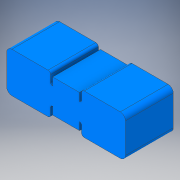
# Autodesk Inventor part: Connecter EM
Saved by Autodesk Inventor 2017 (Build 210142000, 142)
## iProperties
Created: 2020-02-07
Part Number: Connecter EM
Material: ABS Plastic
Document SubType Name: Modeling
Designer: 10042265
Density: 1.06 g/cm^3
Appearance: Smooth - White
Author: 10042265
Autodesk Inventor part; units mm, degrees
ref_plane "YZ Plane" through (0, 0, 0) normal (1, 0, 0) x (0, 1, 0)
ref_plane "XZ Plane" through (0, 0, 0) normal (0, 1, 0) x (-1, 0, 0)
ref_plane "XY Plane" through (0, 0, 0) normal (0, 0, 1) x (1, 0, 0)
sketch "Sketch1" plane through (0, 0, 0) normal (0, 0, 1) x (1, 0, 0)
  line L0 (-29.21, 0) -> (-29.21, 7.366)
  line L1 (-26.67, 9.906) -> (-8.89, 9.906)
  line L2 (-7.62, 8.636) -> (-7.62, 5.334)
  line L3 (-6.604, 4.318) -> (-6.604, 4.318)
  line L4 (-6.604, 4.318) -> (-6.604, 8.128)
  line L5 (-6.604, 8.128) -> (0, 8.128)
  arc A0 (-26.67, 9.906) -> (-29.21, 7.366) centre (-26.67, 7.366) ccw
  arc A1 (-7.62, 8.636) -> (-8.89, 9.906) centre (-8.89, 8.636) ccw
  arc A2 (-7.62, 5.334) -> (-6.604, 4.318) centre (-6.604, 5.334) ccw
  line L6 (29.21, 0) -> (29.21, 7.366)
  line L7 (26.67, 9.906) -> (8.89, 9.906)
  line L8 (7.62, 8.636) -> (7.62, 5.334)
  line L9 (6.604, 4.318) -> (6.604, 4.318)
  line L10 (6.604, 4.318) -> (6.604, 8.128)
  line L11 (6.604, 8.128) -> (0, 8.128)
  arc A3 (29.21, 7.366) -> (26.67, 9.906) centre (26.67, 7.366) ccw
  arc A4 (8.89, 9.906) -> (7.62, 8.636) centre (8.89, 8.636) ccw
  arc A5 (6.604, 4.318) -> (7.62, 5.334) centre (6.604, 5.334) ccw
  line L12 (-29.21, 0) -> (-29.21, -7.366)
  line L13 (-26.67, -9.906) -> (-8.89, -9.906)
  line L14 (-7.62, -8.636) -> (-7.62, -5.334)
  arc A6 (-29.21, -7.366) -> (-26.67, -9.906) centre (-26.67, -7.366) ccw
  arc A7 (-8.89, -9.906) -> (-7.62, -8.636) centre (-8.89, -8.636) ccw
  arc A8 (-6.604, -4.318) -> (-7.62, -5.334) centre (-6.604, -5.334) ccw
  arc A9 (7.62, -5.334) -> (6.604, -4.318) centre (6.604, -5.334) ccw
  arc A10 (7.62, -8.636) -> (8.89, -9.906) centre (8.89, -8.636) ccw
  line L15 (26.67, -9.906) -> (8.89, -9.906)
  arc A11 (26.67, -9.906) -> (29.21, -7.366) centre (26.67, -7.366) ccw
  line L16 (29.21, 0) -> (29.21, -7.366)
  line L17 (7.62, -8.636) -> (7.62, -5.334)
  line L18 (-6.604, -4.318) -> (-6.604, -8.128)
  line L19 (-6.604, -8.128) -> (6.604, -8.128)
  line L20 (6.604, -8.128) -> (6.604, -4.318)
  point P0 (0, 0)
  point P1 (-29.21, 9.906)
  point P2 (-7.62, 9.906)
  point P3 (-7.62, 4.318)
  point P4 (29.21, 9.906)
  point P5 (7.62, 9.906)
  point P6 (7.62, 4.318)
  point P7 (-29.21, -9.906)
  point P8 (-7.62, -9.906)
  point P9 (-7.62, -4.318)
  point P10 (7.62, -4.318)
  point P11 (7.62, -9.906)
  point P12 (29.21, -9.906)
  dimension "d1" = 9.906
  dimension "d2" = 21.59
  dimension "d3" = 5.588
  dimension "d4" = 1.016
  dimension "d5" = 8.128
  dimension "d6" = 2.54
  dimension "d7" = 1.27
  dimension "d8" = 1.016
  constraints: 42 end point, 24 point on circle, 22 point on line, 12 centre point, 6 tangent, 5 perpendicular, 2 horizontal, 1 vertical
  measures "d1" distance of L0.start point (-29.21, 9.906)
  measures "d2" distance of point (-29.21, 9.906) point (-7.62, 9.906)
  measures "d3" distance of point (-7.62, 9.906) point (-7.62, 4.318)
  measures "d4" distance of point (-7.62, 4.318) L3.end
  measures "d5" distance of point (0, 0) L5.end
  measures "d6" radius of A0
  measures "d7" radius of A1
  measures "d8" radius of A2
extrude "Extrusion1" add sketch "Sketch1" along normal blind 23.5204
body "Solid1"
